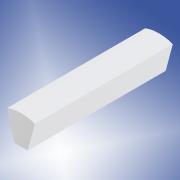
# Autodesk Inventor part: SA001
Saved by Autodesk Inventor 2017 (Build 210142000, 142)
## iProperties
Created: 2017-06-05
Part Number: SA001
Material: ABS Plastic
Document SubType Name: Modeling
Designer: Zach
Density: 1.06 g/cm^3
Appearance: CR White
Author: Zach
Autodesk Inventor part; units mm, degrees
ref_plane "YZ Plane" through (0, 0, 0) normal (1, 0, 0) x (0, 1, 0)
ref_plane "XZ Plane" through (0, 0, 0) normal (0, 1, 0) x (-1, 0, 0)
ref_plane "XY Plane" through (0, 0, 0) normal (0, 0, 1) x (1, 0, 0)
sketch "Sketch3" plane through (0, 0, 0) normal (0, 0, 1) x (1, 0, 0)
  line L0 (0, 0) -> (160, 0)
  line L1 (160, 0) -> (118.589, -154.5481)
  line L2 (0, 0) -> (41.411, -154.5481)
  line L3 (41.411, -154.5481) -> (118.589, -154.5481)
  dimension "d26" = 160
  dimension "d27" = 160
  dimension "d28" = 75
  dimension "d29" = 75
  constraints: 8 end point, 2 horizontal
  measures "d26" distance of L0.start L0.end
  measures "d27" distance of L0.end L1.end
  measures "d28" angle of L0 L1
  measures "d29" angle of L0 L2
extrude "Extrusion3" add sketch "Sketch3" along normal blind 800
sketch "Sketch4" plane through (0, 0, 800) normal (0, 0, 1) x (1, 0, 0)
  circle A0 centre (80, -210.2974) radius 225 construction
  line L0 (160, 0) -> (0, 0) projected
  line L1 (0, 0) -> (160, 0)
  arc A1 (160, 0) -> (0, 0) centre (80, -210.2974) ccw
  dimension "d30" = 450
  constraints: 4 point on circle, 2 centre point, 2 end point, 1 concentric, 1 horizontal
  measures "d30" diameter of A0
extrude "Extrusion4" add sketch "Sketch4" against normal blind 800
body "Solid2"
